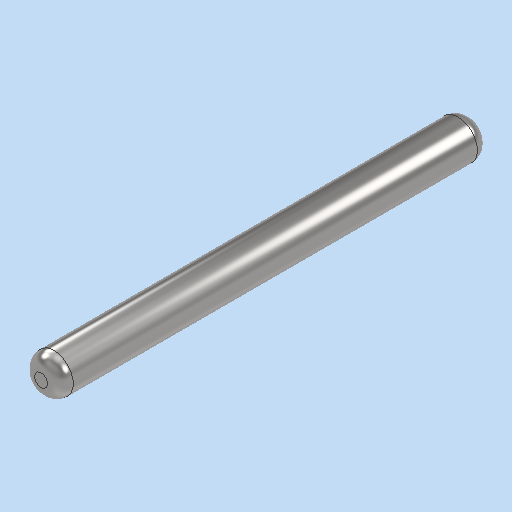
# Autodesk Inventor part: Peça2 - macaco
Saved by Autodesk Inventor 2025.3 (Build 293356000, 356)
## iProperties
Created: 2025-10-09
Part Number: Peça2 - macaco
Material: Aço, carbono
Document SubType Name: Modeling
Designer: gabriel.bispo
Density: 7.85 g/cm^3
Appearance: Semipolido
Author: gabriel.bispo
Autodesk Inventor part; units mm, degrees
ref_plane "YZ Plane" through (0, 0, 0) normal (1, 0, 0) x (0, 1, 0)
ref_plane "XZ Plane" through (0, 0, 0) normal (0, 1, 0) x (-1, 0, 0)
ref_plane "XY Plane" through (0, 0, 0) normal (0, 0, 1) x (1, 0, 0)
sketch "Esboço1" plane through (0, 0, 0) normal (0, 1, 0) x (-1, 0, 0)
  line L0 (0, 48.139) -> (0, -51.861)
  line L1 (0, 48.139) -> (1.5, 48.139)
  line L2 (4.5, 45.139) -> (4.5, -48.861)
  line L3 (1.5, -51.861) -> (0, -51.861)
  arc A0 (4.5, 45.139) -> (1.5, 48.139) centre (1.5, 45.139) ccw
  arc A1 (1.5, -51.861) -> (4.5, -48.861) centre (1.5, -48.861) ccw
  point P0 (0, 0)
  point P1 (0, -1.861)
  point P2 (4.5, 48.139)
  dimension "d0" = 100
  dimension "d1" = 4.5
  dimension "d2" = 3
  constraints: 8 end point, 4 point on circle, 4 tangent, 2 centre point, 2 point on line, 2 vertical, 1 equal radius, 1 horizontal, 1 midpoint, 1 perpendicular, 1 vertical alignment
  measures "d0" distance of L0.start L0.end
  measures "d1" distance of L0.start point (4.5, 48.139)
  measures "d2" radius of A0
revolve "Revolução1" add sketch "Esboço1" angle 360 about axis through (0, 0, 48.139) along (0, 0, -1)
